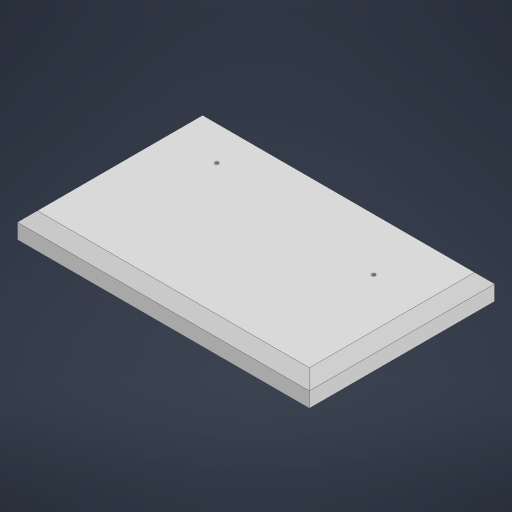
# Autodesk Inventor part: sf_Wood_Base_1
Saved by Autodesk Inventor 2024 (Build 280153000, 153)
## iProperties
Created: 2024-03-20
Part Number: sf_Wood_Base_1
Material: Generisch
Document SubType Name: Modeling
Designer: Simon
Density: 1 g/cm^3
Appearance: Vorgabe
Author: Simon
Autodesk Inventor part; units mm, degrees
ref_plane "YZ Plane" through (0, 0, 0) normal (1, 0, 0) x (0, 1, 0)
ref_plane "XZ Plane" through (0, 0, 0) normal (0, 1, 0) x (-1, 0, 0)
ref_plane "XY Plane" through (0, 0, 0) normal (0, 0, 1) x (1, 0, 0)
sketch "Skizze1" plane through (0, 0, 0) normal (0, 0, 1) x (1, 0, 0)
  line L0 (-87.5, -55.5) -> (87.5, -55.5)
  line L1 (87.5, -55.5) -> (87.5, 55.5)
  line L2 (87.5, 55.5) -> (-87.5, 55.5)
  line L3 (-87.5, 55.5) -> (-87.5, -55.5)
  line L4 (-87.5, -55.5) -> (87.5, 55.5) construction
  line L5 (87.5, -55.5) -> (-87.5, 55.5) construction
  point P0 (0, 0)
  dimension "d0" = 175
  dimension "d1" = 111
  constraints: 12 end point, 2 midpoint, 2 parallel, 1 horizontal, 1 perpendicular
  measures "d0" distance of L2.end L1.end
  measures "d1" distance of L1.end L0.end
extrude "Extrusion1" add sketch "Skizze1" along normal blind 15
sketch "Skizze2" plane through (0, 0, 15) normal (0, 0, 1) x (1, 0, 0)
  line L0 (87.5, 55.5) -> (-87.5, 55.5) projected
  line L1 (-87.5, 55.5) -> (-52.5, 55.5) construction
  line L2 (-52.5, 55.5) -> (-52.5, 29) construction
  line L3 (-52.5, 29) -> (-87.5, 29) construction
  line L4 (-87.5, 29) -> (-87.5, 55.5) construction
  line L5 (87.5, 55.5) -> (52.5, 55.5) construction
  line L6 (52.5, 55.5) -> (52.5, 18) construction
  line L7 (52.5, 18) -> (87.5, 18) construction
  line L8 (87.5, 18) -> (87.5, 55.5) construction
  circle A0 centre (-52.5, 29) radius 1
  circle A1 centre (52.5, 18) radius 1
  point P0 (0, 0)
  dimension "d4" = 35
  dimension "d5" = 26.5
  dimension "d6" = 35
  dimension "d7" = 37.5
  dimension "d8" = 2
  dimension "d9" = 2
  constraints: 16 end point, 4 parallel, 2 centre point, 2 coincident, 2 horizontal, 2 perpendicular
  measures "d4" distance of L2.end L3.end
  measures "d5" distance of L1.end L2.end
  measures "d6" distance of L7.end L6.end
  measures "d7" distance of L6.end L5.end
  measures "d8" diameter of A0
  measures "d9" diameter of A1
extrude "Extrusion2" cut sketch "Skizze2" against normal blind 19.5
chamfer "Fasen1" distance 6 angle 45 4 edges at (-87.5, 0, 15) (0, -55.5, 15) (87.5, 0, 15) (0, 55.5, 15)
